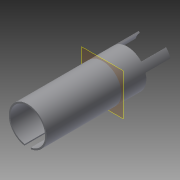
# Autodesk Inventor part: 知能ロボコン大砲１
Saved by Autodesk Inventor 2013 (Build 170138000, 138)
## iProperties
Created: 2014-05-11
Part Number: 知能ロボコン大砲１
Material: 一般
Document SubType Name: Modeling
Designer: horumo136
Density: 1 g/cm^3
Author: horumo136
Autodesk Inventor part; units mm, degrees
ref_plane "YZ Plane" through (0, 0, 0) normal (1, 0, 0) x (0, 1, 0)
ref_plane "XZ Plane" through (0, 0, 0) normal (0, 1, 0) x (-1, 0, 0)
ref_plane "XY Plane" through (0, 0, 0) normal (0, 0, 1) x (1, 0, 0)
sketch "スケッチ1" plane through (0, 0, 0) normal (0, 1, 0) x (-1, 0, 0)
  circle A0 centre (0, 0) radius 35
  circle A1 centre (0, 0) radius 38
  dimension "d0" = 70
  dimension "d1" = 76
  constraints: 2 centre point, 2 coincident
  measures "d0" diameter of A0
  measures "d1" diameter of A1
extrude "押し出し1" add sketch "スケッチ1" along normal blind 250
sketch "スケッチ2" plane through (0, 250, 0) normal (0, 1, 0) x (1, 0, 0)
  circle A0 centre (0, 0) radius 38 projected
  line L0 (0, 0) -> (-27.1351, -26.6024)
  line L1 (0, 0) -> (27.9749, -25.7178)
  line L2 (0, 0) -> (-27.1351, -26.6024)
  circle A1 centre (0, 0) radius 35 projected
  line L3 (0, 0) -> (-36.4384, -10.7818)
  line L4 (0, 0) -> (36.4384, -10.7818)
  point P0 (-32.2602, -20.0818)
  point P1 (33.0208, -18.805)
  constraints: 10 end point, 8 other
extrude "押し出し3" cut sketch "スケッチ2" against normal blind 50 contours A0 L4 A1 L3 | L0 A1 L1 A0 | A1 L4 L3 | L0 L1 A1
ref_plane "作業平面2" through (0, 150, 0) normal (0, -1, 0) x (1, 0, 0)
sketch "スケッチ3" plane through (0, 150, 0) normal (0, -1, 0) x (1, 0, 0)
  circle A0 centre (0, 0) radius 35
  circle A1 centre (0, 0) radius 30
  dimension "d10" = 70
  dimension "d11" = 60
  constraints: 2 centre point, 2 coincident
  measures "d10" diameter of A0
  measures "d11" diameter of A1
extrude "押し出し4" add sketch "スケッチ3" against normal blind 5
sketch "スケッチ4" plane through (0, 0, 0) normal (0, -1, 0) x (1, 0, 0)
  circle A0 centre (0, 0) radius 38 projected
  line L0 (0, 0) -> (6.5986, -37.4227)
  line L1 (0, 0) -> (38, 0) construction
  line L2 (0, 0) -> (-6.5986, -37.4227)
  line L3 (0, 0) -> (38, 0) construction
  dimension "d14" = 80
  dimension "d15" = 100
  constraints: 8 end point, 2 equal length, 2 horizontal, 2 point on circle
  measures "d14" angle of L0 L1
  measures "d15" angle of L2 L3
extrude "押し出し5" cut sketch "スケッチ4" against normal blind 50 contours L2 L0 A0 picked at (0, -25.2905)
